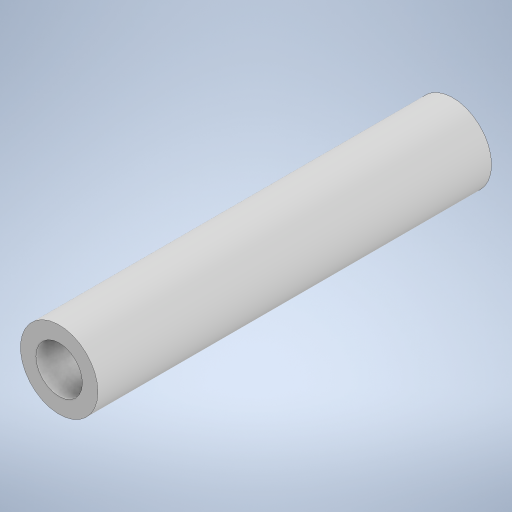
# Autodesk Inventor part: prenetration_top_sweep
Saved by Autodesk Inventor 2023 (Build 270158000, 158)
## iProperties
Created: 2023-01-25
Part Number: prenetration_top_sweep
Material: Generic
Document SubType Name: Modeling
Designer: remidm
Density: 1 g/cm^3
Appearance: Default
Mass: 0.506707 g
Surface Area: 10.5331 cm^2
Volume: 0.506707 cm^3
PenetrationOuterDiameter: 0.197 in
Author: remidm
Autodesk Inventor part; units mm, degrees
ref_plane "YZ Plane" through (0, 0, 0) normal (1, 0, 0) x (0, 1, 0)
ref_plane "XZ Plane" through (0, 0, 0) normal (0, 1, 0) x (-1, 0, 0)
ref_plane "XY Plane" through (0, 0, 0) normal (0, 0, 1) x (1, 0, 0)
sketch "Sketch1" plane through (0, 0, 0) normal (0, 0, 1) x (1, 0, 0)
  circle A0 centre (0, 0) radius 2.5
  dimension "PenetrationOuterDiameter" = 5
  constraints: 1 centre point
  measures "PenetrationOuterDiameter" diameter of A0
extrude "Extrusion2" add sketch "Sketch1" along normal blind 25.4
hole "Hole2" at (0, 0, 0) direction (0, 0, 1) diameter 3 end through all
equation "\"PenetrationInnerDiameter\" = PenetrationOuterDiameter - 2 * PenetrationThickness"
equation "\"PenetrationThickness\" = 1"
body "Solid2"
